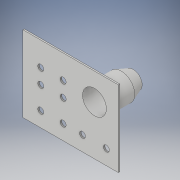
# Autodesk Inventor part: OpeningV2
Saved by Autodesk Inventor 2019 (Build 230136000, 136)
## iProperties
Created: 2020-09-08
Part Number: OpeningV2
Material: Generic
Document SubType Name: Modeling
Designer: ASUS
Density: 1 g/cm^3
Appearance: Default
Author: ASUS
Autodesk Inventor part; units mm, degrees
ref_plane "YZ Plane" through (0, 0, 0) normal (1, 0, 0) x (0, 1, 0)
ref_plane "XZ Plane" through (0, 0, 0) normal (0, 1, 0) x (-1, 0, 0)
ref_plane "XY Plane" through (0, 0, 0) normal (0, 0, 1) x (1, 0, 0)
sketch "Sketch1" plane through (0, 0, 0) normal (0, 0, 1) x (1, 0, 0)
  line L0 (-48, 18) -> (16, 18)
  line L1 (16, 18) -> (16, -33)
  line L2 (16, -33) -> (-48, -33)
  line L3 (-48, -33) -> (-48, 18)
  circle A0 centre (0, 0) radius 8
  dimension "d0" = 64
  dimension "d1" = 51
  dimension "d2" = 18
  dimension "d3" = 16
  dimension "d4" = 16
  constraints: 8 end point, 2 parallel, 1 centre point, 1 coincident, 1 horizontal, 1 perpendicular
  measures "d0" distance of L0.start L0.end
  measures "d1" distance of L0.end L1.end
  measures "d2" distance from line of L0 point (0, 0)
  measures "d3" distance from line of L1 point (0, 0)
  measures "d4" diameter of A0
extrude "Extrusion1" add sketch "Sketch1" along normal blind 1
sketch "Sketch2" plane through (0, 0, 1) normal (0, 0, 1) x (1, 0, 0)
  line L0 (-48, 18) -> (-48, -33) projected
  line L1 (-48, -33) -> (16, -33) projected
  point P0 (0, 0)
  point P1 (-36, 2)
  point P2 (-36, -8)
  point P3 (-36, -23)
  point P4 (-21, 2)
  point P5 (-21, -8)
  point P6 (-21, -23)
  point P7 (-8, -23)
  point P8 (8, -23)
  dimension "d7" = 12
  dimension "d8" = 15
  dimension "d9" = 13
  dimension "d10" = 16
  dimension "d11" = 10
  dimension "d12" = 15
  dimension "d13" = 10
  constraints: 5 horizontal alignment, 4 vertical alignment
  measures "d7" distance from line of L0 point (-36, -23)
  measures "d8" distance of point (-21, -23) point (-36, -23)
  measures "d9" distance of point (-8, -23) point (-21, -23)
  measures "d10" distance of point (8, -23) point (-8, -23)
  measures "d11" distance from line of L1 point (-36, -23)
  measures "d12" distance of point (-36, -8) point (-36, -23)
  measures "d13" distance of point (-36, 2) point (-36, -8)
hole "Hole1" at (-36, 2, 1) at (-36, -8, 1) at (-36, -23, 1) at (-21, 2, 1) at (-21, -8, 1) at (-21, -23, 1) at (-8, -23, 1) at (8, -23, 1) direction (0, 0, -1) diameter 4 end through all
sketch "Sketch7" plane through (0, 0, 0) normal (1, 0, 0) x (0, 1, 0)
  line L0 (8, 0) -> (-8, 0) projected
  line L1 (5, -25) -> (6, -25)
  line L2 (18, 0) -> (-33, 0) projected
  line L3 (8, 0) -> (9, 0)
  line L4 (0, -31.2) -> (0, 5.2) projected
  line L5 (9, 0) -> (9, -17)
  line L6 (9, -17) -> (6, -25)
  line L7 (8, 0) -> (8, -17)
  line L8 (8, -17) -> (5, -25)
  point P0 (0, 0)
  dimension "d33" = 25
  dimension "d34" = 1
  dimension "d35" = 5
  dimension "d37" = 17
  constraints: 12 end point, 3 parallel, 2 vertical, 1 horizontal alignment, 1 point on line
  measures "d33" vertical distance of L1.end L0.start
  measures "d34" distance of L1.start L1.end
  measures "d35" horizontal distance of point (0, 0) L1.start
  measures "d37" distance of L3.end L5.end
revolve "Revolution1" add sketch "Sketch7" angle 360 about axis through (0, 0, -10) along (0, 0, 1)
sketch "Sketch8" plane through (0, 0, -25) normal (0, 0, -1) x (-1, 0, 0)
  point P0 (0, 0)
body "Solid1"
